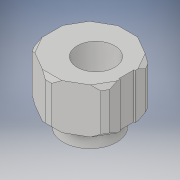
# Autodesk Inventor part: Eccentric Spacer
Saved by Autodesk Inventor 2019 (Build 230136000, 136)
## iProperties
Created: 2021-03-24
Part Number: Eccentric Spacer
Material: Generic
Document SubType Name: Modeling
Designer: asus
Density: 1 g/cm^3
Appearance: Default
Author: asus
Autodesk Inventor part; units mm, degrees
ref_plane "YZ Plane" through (0, 0, 0) normal (1, 0, 0) x (0, 1, 0)
ref_plane "XZ Plane" through (0, 0, 0) normal (0, 1, 0) x (-1, 0, 0)
ref_plane "XY Plane" through (0, 0, 0) normal (0, 0, 1) x (1, 0, 0)
sketch "Sketch1" plane through (0, 0, 0) normal (0, 1, 0) x (-1, 0, 0)
  line L0 (-4.567, 3.1368) -> (-0.433, 5.5235)
  line L1 (0.433, 5.5235) -> (4.567, 3.1368)
  line L2 (5, 2.3868) -> (5, -2.3868)
  line L3 (4.567, -3.1368) -> (0.433, -5.5235)
  line L4 (-0.433, -5.5235) -> (-4.567, -3.1368)
  circle A0 centre (0, 0) radius 3.555
  circle A1 centre (-0.79, 0) radius 2.5
  line L5 (0.433, 5.5235) -> (-0.433, 5.5235)
  line L6 (-4.567, 3.1368) -> (-5, 2.3868)
  line L7 (4.567, 3.1368) -> (5, 2.3868)
  line L8 (5, -2.3868) -> (4.567, -3.1368)
  line L9 (0.433, -5.5235) -> (-0.433, -5.5235)
  line L10 (-4.567, -3.1368) -> (-5, -2.3868)
  line L11 (-5, -1) -> (-4.85, -1)
  line L12 (-4.85, -1) -> (-4.85, 1)
  line L13 (-4.85, 1) -> (-5, 1)
  line L14 (-5, -2.3868) -> (-5, -1)
  line L15 (-5, 1) -> (-5, 2.3868)
  point P0 (-5, 2.8868)
  point P1 (0, 5.7735)
  point P2 (5, 2.8868)
  point P3 (5, -2.8868)
  point P4 (0, -5.7735)
  point P5 (-5, -2.8868)
  point P6 (-4.85, 0)
  dimension "d1" = 7.11
  dimension "d2" = 5
  dimension "d3" = 0.79
  dimension "d4" = 0.5
  dimension "d5" = 0.5
  dimension "d6" = 0.5
  dimension "d7" = 0.5
  dimension "d8" = 0.5
  dimension "d9" = 0.5
  dimension "d10" = 0.5
  dimension "d11" = 0.5
  dimension "d12" = 0.5
  dimension "d13" = 0.5
  dimension "d14" = 0.5
  dimension "d15" = 0.5
  dimension "d16" = 2
  constraints: 32 end point, 10 point on line, 2 centre point, 2 coincident, 2 horizontal alignment, 1 horizontal, 1 midpoint, 1 parallel, 1 perpendicular, 11 other
  measures "d1" diameter of A0
  measures "d2" diameter of A1
  measures "d3" distance of point (0, 0) A1.centre
  measures "d4" distance of L1.start point (0, 5.774)
  measures "d5" distance of L0.end point (0, 5.774)
  measures "d6" distance of L0.start point (-5, 2.887)
  measures "d7" distance of L6.end point (-5, 2.887)
  measures "d8" distance of L1.end point (5, 2.887)
  measures "d9" distance of L2.start point (5, 2.887)
  measures "d10" distance of L2.end point (5, -2.887)
  measures "d11" distance of L3.start point (5, -2.887)
  measures "d12" distance of L3.end point (0, -5.774)
  measures "d13" distance of L4.start point (0, -5.774)
  measures "d14" distance of L4.end point (-5, -2.887)
  measures "d15" distance of L10.end point (-5, -2.887)
  measures "d16" distance of L11.end L12.end
extrude "Extrusion1" add sketch "Sketch1" along normal blind 6 contours L0 L5 L1 L7 L2 L8 L3 L9 L4 L10 L14 L11 L12 L13 L15 L6 | A0
extrude "Extrusion2" add sketch "Sketch1" against normal blind 2.5 contours A0
chamfer "Chamfer1" distance 0.5 angle 45 12 edges at (-4.7835, 0, -2.7618) (0, 0, -5.5235) (-4.7835, 0, 2.7618) (4.7835, 0, -2.7618) (4.7835, 0, 2.7618) (0, 0, 5.5235) (4.7835, 6, 2.7618) (0, 6, 5.5235) (-4.7835, 6, 2.7618) (-4.7835, 6, -2.7618) (0, 6, -5.5235) (4.7835, 6, -2.7618)
equation "\"d5\" = d4"
equation "\"d6\" = d4"
equation "\"d7\" = d6"
equation "\"d8\" = d4"
equation "\"d9\" = d8"
equation "\"d10\" = d4"
equation "\"d11\" = d10"
equation "\"d12\" = d4"
equation "\"d13\" = d12"
equation "\"d14\" = d4"
equation "\"d15\" = d14"
body "Solid1"
